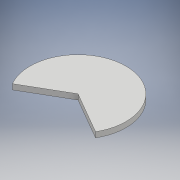
# Autodesk Inventor part: RescueKitThrow-Jointv2
Saved by Autodesk Inventor 2018.3 (Build 223284000, 284)
## iProperties
Created: 2019-03-13
Part Number: RescueKitThrow-Jointv2
Material: 一般
Document SubType Name: Modeling
Designer: shun2
Density: 1 g/cm^3
Appearance: 既定
Author: shun2
Autodesk Inventor part; units mm, degrees
ref_plane "YZ Plane" through (0, 0, 0) normal (1, 0, 0) x (0, 1, 0)
ref_plane "XZ Plane" through (0, 0, 0) normal (0, 1, 0) x (-1, 0, 0)
ref_plane "XY Plane" through (0, 0, 0) normal (0, 0, 1) x (1, 0, 0)
sketch "スケッチ1" plane through (0, 0, 0) normal (0, 0, 1) x (1, 0, 0)
  arc A0 (38.9711, -22.5) -> (-38.9711, -22.5) centre (0, 0) ccw
  line L0 (0, 0) -> (-38.9711, -22.5)
  line L1 (0, 0) -> (45, 0) construction
  line L2 (0, 0) -> (38.9711, -22.5)
  line L3 (0, 0) -> (45, 0) construction
  dimension "d0" = 90
  dimension "d1" = 150
  dimension "d2" = 330
  constraints: 8 end point, 2 equal length, 2 horizontal, 2 point on circle, 1 centre point, 1 coincident
  measures "d0" diameter of A0
  measures "d1" angle of L0 L1
extrude "押し出し1" add sketch "スケッチ1" along normal blind 5
